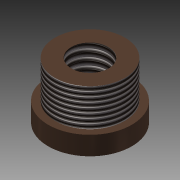
# Autodesk Inventor part: ACME Threaded Rod Nut
Saved by Autodesk Inventor 2013 (Build 170138000, 138)
## iProperties
Created: 2013-01-17
Part Number: ACME Threaded Rod Nut
Material: Bronze, Cast
Document SubType Name: Modeling
Designer: actoennies
Density: 8.87 g/cm^3
Mass: 64.5101 g
Surface Area: 32.9502 cm^2
Volume: 7.27285 cm^3
Author: actoennies
Autodesk Inventor part; units mm, degrees
ref_plane "YZ Plane" through (0, 0, 0) normal (1, 0, 0) x (0, 1, 0)
ref_plane "XZ Plane" through (0, 0, 0) normal (0, 1, 0) x (-1, 0, 0)
ref_plane "XY Plane" through (0, 0, 0) normal (0, 0, 1) x (1, 0, 0)
sketch "Sketch1" plane through (0, 0, 0) normal (0, 1, 0) x (-1, 0, 0)
  circle A0 centre (0, 0) radius 14.224
  dimension "d0" = 28.448
  constraints: 1 centre point, 1 coincident
  measures "d0" diameter of A0
extrude "Extrusion1" add sketch "Sketch1" along normal blind 6.35
sketch "Sketch2" plane through (0, 6.35, 0) normal (0, 1, 0) x (1, 0, 0)
  circle A0 centre (0, 0) radius 14.224 projected
  circle A1 centre (0, 0) radius 11.8999
  dimension "d3" = 23.7998
  constraints: 1 centre point, 1 coincident
  measures "d3" diameter of A1
extrude "Extrusion2" add sketch "Sketch2" along normal blind 12.7 contours A1
sketch "Sketch3" plane through (0, 19.05, 0) normal (0, 1, 0) x (1, 0, 0)
  circle A0 centre (0, 0) radius 11.8999 projected
  circle A1 centre (0, 0) radius 6.35
  dimension "d6" = 12.7
  constraints: 1 centre point, 1 coincident
  measures "d6" diameter of A1
extrude "Extrusion3" cut sketch "Sketch3" against normal blind 2540 contours A1
thread "Thread1" size "15/16-16 UN" class "2A" standard "ANSI Unified Screw Threads" full length
thread "Thread2" size "1-10 UNS" class "2B" standard "ANSI Unified Screw Threads" full length
body "Solid1"
